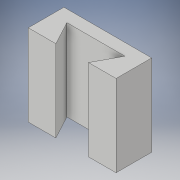
# Autodesk Inventor part: Schienenläuderaufsatz_22.5
Saved by Autodesk Inventor 2018.3 (Build 223284000, 284)
## iProperties
Created: 2018-10-11
Part Number: Schienenläuderaufsatz_22.5
Material: Generisch
Document SubType Name: Modeling
Designer: pgmadmin
Density: 1 g/cm^3
Appearance: Vorgabe
Author: pgmadmin
Autodesk Inventor part; units mm, degrees
ref_plane "YZ Plane" through (0, 0, 0) normal (1, 0, 0) x (0, 1, 0)
ref_plane "XZ Plane" through (0, 0, 0) normal (0, 1, 0) x (-1, 0, 0)
ref_plane "XY Plane" through (0, 0, 0) normal (0, 0, 1) x (1, 0, 0)
sketch "Skizze1" plane through (0, 0, 0) normal (0, 0, 1) x (1, 0, 0)
  line L0 (-18.6218, 0) -> (-22.9018, 8)
  line L1 (-22.9018, 8) -> (-3.3418, 8)
  line L2 (-3.3418, 8) -> (-7.6218, 0)
  line L3 (-7.6218, 0) -> (-18.6218, 0)
  line L4 (-18.6218, 0) -> (-27.9018, 0)
  line L5 (-27.9018, 0) -> (-27.9018, 12)
  line L6 (-27.9018, 12) -> (1.6582, 12)
  line L7 (1.6582, 12) -> (1.6582, 0)
  line L8 (1.6582, 0) -> (-7.6218, 0)
  point P0 (0, 0)
  dimension "d0" = 8
  dimension "d1" = 11
  dimension "d3" = 4.28
  dimension "d6" = 4.28
  dimension "d7" = 4
  dimension "d8" = 5
  dimension "d9" = 5
  dimension "d10" = 29.56
  constraints: 18 end point, 4 perpendicular, 2 horizontal, 1 parallel, 1 point on line
  measures "d0" vertical distance of L0.start L0.end
  measures "d1" distance of L2.end L0.start
  measures "d3" horizontal distance of L0.end L0.start
  measures "d6" horizontal distance of L1.end L2.end
  measures "d7" distance between parallel lines of L6 L1
  measures "d8" distance from line of L5 L0.end
  measures "d9" distance from line of L7 L1.end
  measures "d10" distance of L5.end L6.end
extrude "Extrusion1" add sketch "Skizze1" along normal blind 27.5 contours L4 L5 L6 L7 L8 L2 L1 L0
